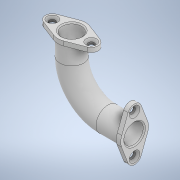
# Autodesk Inventor part: Część14
Saved by Autodesk Inventor 2021 (Build 250183000, 183)
## iProperties
Created: 2023-10-11
Part Number: Część14
Material: Ogólny
Document SubType Name: Modeling
Designer: Jakub
Density: 1 g/cm^3
Appearance: Domyślna
Author: Jakub
Autodesk Inventor part; units mm, degrees
ref_plane "YZ Plane" through (0, 0, 0) normal (1, 0, 0) x (0, 1, 0)
ref_plane "XZ Plane" through (0, 0, 0) normal (0, 1, 0) x (-1, 0, 0)
ref_plane "XY Plane" through (0, 0, 0) normal (0, 0, 1) x (1, 0, 0)
sketch "Szkic1" plane through (0, 0, 0) normal (0, 1, 0) x (-1, 0, 0)
  circle A0 centre (0, 0) radius 25
  line L0 (0, 0) -> (-35, 0)
  line L1 (-35, 0) -> (35, 0)
  circle A1 centre (35, 0) radius 12.5
  circle A2 centre (-35, 0) radius 12.5
  line L2 (35, -12.5) -> (9.6154, -23.0769)
  line L3 (9.6154, -23.0769) -> (39.4603, -11.6771)
  line L4 (9.6154, 23.0769) -> (39.4603, 11.6771)
  line L5 (-9.6154, -23.0769) -> (-39.4603, -11.6771)
  line L6 (-39.4603, 11.6771) -> (-8.2178, 23.6108)
  point P0 (24.1964, 6.2875)
  point P1 (24.1964, -6.2875)
  dimension "d0" = 50
  dimension "d1" = 35
  dimension "d2" = 70
  dimension "d3" = 25
  dimension "d4" = 25
  constraints: 14 end point, 9 point on circle, 5 tangent, 3 centre point, 3 coincident, 1 horizontal, 1 parallel, 1 point on line
  measures "d0" diameter of A0
  measures "d1" distance of L0.start L0.end
  measures "d2" distance of L0.end L1.end
  measures "d3" diameter of A1
  measures "d4" diameter of A2
extrude "Wyciągnięcie proste1" add sketch "Szkic1" along normal blind 8 contours A0 A1 L1 L0 A2 L6 | L4 A1 A0 | A1 A0 | A0 L1 A1 | A0 A2 L6 | A0 A1 L1 | A1 A0 A2 L0 L1 | A2 L0 A0 | A0 A2 | A1 L2 A0 | L3 L2 A1 | L0 A2 A0 | A2 A0 L5
sketch "Szkic2" plane through (0, 8, 0) normal (0, 1, 0) x (1, 0, 0)
  circle A0 centre (0, 0) radius 20
  circle A1 centre (0, 0) radius 17.5
  dimension "d7" = 40
  dimension "d8" = 35
  constraints: 2 centre point, 2 coincident
  measures "d7" diameter of A0
  measures "d8" diameter of A1
extrude "Wyciągnięcie proste2" cut sketch "Szkic2" against normal blind 8 contours A1
chamfer "Faza1" distance 2 angle 45 1 edges at (-17.5, 8, 0)
sketch "Szkic4" plane through (0, 8, 0) normal (0, 1, 0) x (1, 0, 0)
  circle A0 centre (-35, 0) radius 5.5
  circle A1 centre (35, 0) radius 5.5
  point P0 (0, 0)
  dimension "d15" = 11
  dimension "d16" = 11
  constraints: 2 centre point
  measures "d15" diameter of A0
  measures "d16" diameter of A1
extrude "Wyciągnięcie proste3" cut sketch "Szkic4" against normal blind 8
chamfer "Faza2" distance 4 angle 45 2 edges at (-40.5, 8, 0) (29.5, 8, 0)
sketch "Szkic6" plane through (0, 0, 0) normal (0, 0, 1) x (1, 0, 0)
  line L0 (0, 0) -> (-21.5, 0)
  line L1 (9.6154, 0) -> (-9.6154, 0) projected
  line L2 (-21.5, 0) -> (21.5, 0)
  line L3 (8.2178, 0) -> (39.4603, 0) projected
  line L4 (-47.5, 0) -> (-47.5, 8) projected
  line L5 (-47.5, 8) -> (-47.5, -144.5)
  line L6 (21.5, 0) -> (21.5, -32)
  line L7 (21.5, -144.5) -> (-47.5, -144.5)
  line L8 (-47.5, -144.5) -> (105, -144.5)
  line L9 (-21.5, 0) -> (-21.5, -32)
  line L10 (-39.4603, 0) -> (-9.6154, 0) projected
  line L11 (105, -144.5) -> (105, -118.5)
  line L12 (105, -118.5) -> (65, -118.5)
  line L13 (105, -118.5) -> (105, -75.5)
  line L14 (105, -75.5) -> (65, -75.5)
  arc A0 (21.5, -32) -> (65, -75.5) centre (65, -32) ccw
  arc A1 (-21.5, -32) -> (65, -118.5) centre (65, -32) ccw
  point P0 (-21.5, -144.5)
  dimension "d24" = 21.5
  dimension "d25" = 43
  dimension "d26" = 152.5
  dimension "d28" = 152.5
  dimension "d30" = 26
  dimension "d31" = 43
  dimension "d32" = 43.5
  dimension "d33" = 86.5
  constraints: 22 end point, 7 point on line, 4 point on circle, 4 tangent, 2 centre point, 2 collinear, 2 perpendicular, 2 vertical
  measures "d24" distance of L0.start L0.end
  measures "d25" distance of L0.end L2.end
  measures "d26" distance of L5.start L5.end
  measures "d28" distance of L5.end L8.end
  measures "d30" distance of L8.end L11.end
  measures "d31" distance of L11.end L13.end
  measures "d32" radius of A0
  measures "d33" radius of A1
extrude "Wyciągnięcie proste4" [suppressed]
fillet "Zaokrąglenie1" [suppressed]
sketch "Szkic7" plane through (105, -97, 0) normal (1, 0, 0) x (0, 1, 0)
  circle A0 centre (0, 0) radius 25
  line L0 (0, 0) -> (-35, 0)
  line L1 (-35, 0) -> (35, 0)
  circle A1 centre (35, 0) radius 12.5
  circle A2 centre (-35, 0) radius 12.5
  line L2 (35, -12.5) -> (9.6154, -23.0769)
  line L3 (9.6154, -23.0769) -> (39.4603, -11.6771)
  line L4 (9.6154, 23.0769) -> (39.4603, 11.6771)
  line L5 (-9.6154, -23.0769) -> (-39.4603, -11.6771)
  line L6 (-39.4603, 11.6771) -> (-8.2178, 23.6108)
  point P0 (24.1964, 6.2875)
  point P1 (24.1964, -6.2875)
  dimension "d41" = 50
  dimension "d40" = 35
  dimension "d39" = 70
  dimension "d38" = 25
  dimension "d37" = 25
  constraints: 14 end point, 9 point on circle, 5 tangent, 3 centre point, 3 coincident, 1 horizontal, 1 parallel, 1 point on line
  measures "d41" diameter of A0
  measures "d40" distance of L0.start L0.end
  measures "d39" distance of L0.end L1.end
  measures "d38" diameter of A1
  measures "d37" diameter of A2
extrude "Wyciągnięcie proste5" [suppressed]
sketch "Szkic8" plane through (0, 0, 0) normal (0, 0, 1) x (1, 0, 0)
  line L0 (17.5, 0) -> (-17.5, 0) projected
  line L1 (0, 0) -> (17.5, 0)
  line L2 (17.5, 0) -> (-17.5, 0)
  line L3 (-39.4603, 0) -> (-9.6154, 0) projected
  line L4 (47.8218, -144.5) -> (-104.6782, -144.5)
  line L5 (0, 0) -> (-21.5, 0)
  line L6 (-47.5, 0) -> (-47.5, 8) projected
  line L7 (-47.5, 8) -> (-47.5, -144.5)
  line L8 (-17.5, 0) -> (-17.5, -44)
  line L9 (-21.5, 0) -> (-21.5, -32)
  line L10 (9.6154, 0) -> (-9.6154, 0) projected
  line L11 (9.6154, 0) -> (9.6154, -144.5)
  line L12 (17.5, 0) -> (17.5, -36)
  line L13 (-47.5, -144.5) -> (105, -144.5)
  line L14 (105, -144.5) -> (105, -118.5)
  line L15 (105, -118.5) -> (105, -75.5)
  line L16 (105, -75.5) -> (65, -75.5)
  line L17 (105, -97) -> (105, -79.5)
  line L18 (105, -79.5) -> (61, -79.5)
  line L19 (105, -97) -> (105, -114.5)
  line L20 (105, -114.5) -> (9.6154, -114.5)
  line L21 (105, -118.5) -> (65, -118.5)
  line L22 (9.6154, -114.5) -> (53, -114.5)
  line L23 (61, -79.5) -> (53, -79.5)
  line L24 (17.5, -44) -> (17.5, -36)
  line L25 (0, 0) -> (21.5, 0)
  line L26 (8.2178, 0) -> (39.4603, 0) projected
  line L27 (21.5, 0) -> (21.5, -32)
  arc A0 (21.5, -32) -> (65, -75.5) centre (65, -32) ccw
  arc A1 (-21.5, -32) -> (65, -118.5) centre (65, -32) ccw
  line L28 (-21.5, -32) -> (-17.5, -32)
  line L29 (-47.5, -144.5) -> (156.8539, -144.5) construction
  line L30 (3.8353, -93.1647) -> (6.6637, -90.3363)
  line L31 (34.2409, -62.7591) -> (31.4124, -65.5876)
  line L32 (-17.5, -44) -> (-17.5, -32)
  line L33 (65, -114.5) -> (9.6154, -114.5)
  line L34 (53, -79.5) -> (65, -79.5)
  line L35 (17.5, -32) -> (17.5, -44)
  arc A2 (17.5, -32) -> (65, -79.5) centre (65, -32) ccw
  arc A3 (-17.5, -32) -> (65, -114.5) centre (65, -32) ccw
  point P0 (-17.5, -144.5)
  point P1 (-21.5, -144.5)
  point P2 (17.5, -144.5)
  point P3 (-17.5, -114.5)
  dimension "d45" = 35
  dimension "d47" = 152.5
  dimension "d50" = 21.5
  dimension "d51" = 152.5
  dimension "d52" = 26
  dimension "d53" = 43
  dimension "d54" = 17.5
  dimension "d55" = 17.5
  dimension "d59" = 21.5
  dimension "d61" = 86.5
  dimension "d63" = 4
  dimension "d64" = 4
  dimension "d65" = 47.5
  dimension "d66" = 82.5
  constraints: 62 end point, 23 point on line, 13 perpendicular, 10 point on circle, 8 tangent, 4 centre point, 3 collinear, 3 horizontal, 1 midpoint, 1 vertical
  measures "d45" distance of L0.start L2.end
  measures "d47" distance of L4.start L4.end
  measures "d50" distance of L1.start L5.end
  measures "d51" distance of L7.end L13.end
  measures "d52" distance of L13.end L14.end
  measures "d53" distance of L14.end L15.end
  measures "d54" distance of L17.start L17.end
  measures "d55" distance of L17.start L19.end
  measures "d59" distance of L1.start L25.end
  measures "d61" radius of A1
  measures "d63" distance of L30.start L30.end
  measures "d64" distance of L31.start L31.end
  measures "d65" radius of A2
  measures "d66" radius of A3
extrude "Wyciągnięcie proste6" add sketch "Szkic8" along normal mid plane 35 contours L25 L27 A0 L31 A2 L12 | A3 L20 A1 L11 | L11 A1 L30 A3 | L31 A0 L16 L15 L18 A2 | L30 A1 L28 A3 | L20 L15 L21 A1 | L28 L9 L3 L8
sketch "Szkic10" plane through (0, 0, 17.5) normal (0, 0, 1) x (1, 0, 0)
  line L0 (-21.5, 0) -> (-21.5, -32) projected
  line L1 (-21.5, 0) -> (-21.5, -32)
  line L2 (105, -118.5) -> (105, -114.5) projected
  line L3 (105, -118.5) -> (65, -118.5)
  line L4 (105, -75.5) -> (65, -75.5)
  line L5 (21.5, 0) -> (21.5, -32) projected
  line L6 (21.5, 0) -> (21.5, -32)
  line L7 (65, -118.5) -> (105, -118.5) projected
  line L8 (105, -75.5) -> (105, -118.5)
  line L9 (21.5, 0) -> (-21.5, 0)
  line L10 (-39.4603, 0) -> (-9.6154, 0) projected
  arc A0 (-21.5, -32) -> (65, -118.5) centre (65, -32) ccw
  arc A1 (21.5, -32) -> (65, -75.5) centre (65, -32) ccw
  point P0 (0, 0)
  dimension "d71" = 86.5
  dimension "d72" = 43.5
  constraints: 12 end point, 4 point on circle, 4 tangent, 2 centre point, 2 collinear, 2 perpendicular, 1 horizontal, 1 vertical
  measures "d71" radius of A0
  measures "d72" radius of A1
extrude "Wyciągnięcie proste7" add sketch "Szkic10" along normal blind 4
sketch "Szkic13" plane through (0, 0, -17.5) normal (0, 0, -1) x (-1, 0, 0)
  line L0 (9.6154, 0) -> (39.4603, 0) projected
  line L1 (-21.5, 0) -> (-21.5, -32) projected
  line L2 (21.447, 0) -> (-21.5, 0)
  line L3 (-65, -75.5) -> (-105, -75.5) projected
  line L4 (-105, -118.5) -> (-65, -118.5) projected
  line L5 (-105, -75.5) -> (-105, -118.5)
  line L6 (-105, -118.5) -> (-65, -118.5)
  line L7 (21.5, -32) -> (21.5, 0) projected
  line L8 (21.5, 0) -> (21.5, -32)
  line L9 (-21.5, 0) -> (-21.5, -32)
  line L10 (-105, -75.5) -> (-65, -75.5)
  arc A0 (-65, -75.5) -> (-21.5, -32) centre (-65, -32) ccw
  arc A1 (-65, -118.5) -> (21.5, -32) centre (-65, -32) ccw
  point P0 (0, 0)
  point P1 (-21.5, -75.5)
  dimension "d75" = 43.5
  dimension "d76" = 86.5
  constraints: 12 end point, 4 point on circle, 4 point on line, 4 tangent, 2 centre point, 2 perpendicular, 2 vertical, 1 collinear
  measures "d75" radius of A0
  measures "d76" radius of A1
extrude "Wyciągnięcie proste8" add sketch "Szkic13" along normal blind 4
fillet "Zaokrąglenie2" radius 17.5 12 edges at (31.4124, -65.5876, -17.5) (17.5, -16, -17.5) (85, -79.5, -17.5) (6.6637, -90.3363, -17.5) (-17.5, -16, -17.5) (85, -114.5, -17.5) (6.6637, -90.3363, 17.5) (-17.5, -16, 17.5) (85, -114.5, 17.5) (31.4124, -65.5876, 17.5) (17.5, -16, 17.5) (85, -79.5, 17.5)
fillet "Zaokrąglenie3" radius 21.5 12 edges at (85, -75.5, -21.5) (34.2409, -62.7591, -21.5) (21.5, -16, -21.5) (3.8353, -93.1647, -21.5) (-21.5, -16, -21.5) (85, -118.5, -21.5) (3.8353, -93.1647, 21.5) (-21.5, -16, 21.5) (85, -118.5, 21.5) (34.2409, -62.7591, 21.5) (21.5, -16, 21.5) (85, -75.5, 21.5)
sketch "Szkic14" plane through (105, -97, 0) normal (1, 0, 0) x (0, 1, 0)
  circle A0 centre (0, 0) radius 25
  line L0 (0, 0) -> (-35, 0)
  line L1 (-35, 0) -> (35, 0)
  circle A1 centre (35, 0) radius 12.5
  circle A2 centre (-35, 0) radius 12.5
  line L2 (35, -12.5) -> (9.6154, -23.0769)
  line L3 (9.6154, -23.0769) -> (39.4603, -11.6771)
  line L4 (9.6154, 23.0769) -> (39.4603, 11.6771)
  line L5 (-9.6154, -23.0769) -> (-39.4603, -11.6771)
  line L6 (-39.4603, 11.6771) -> (-8.2178, 23.6108)
  point P0 (24.1964, 6.2875)
  point P1 (24.1964, -6.2875)
  dimension "d85" = 50
  dimension "d84" = 35
  dimension "d83" = 70
  dimension "d82" = 25
  dimension "d81" = 25
  constraints: 14 end point, 9 point on circle, 5 tangent, 3 centre point, 3 coincident, 1 horizontal, 1 parallel, 1 point on line
  measures "d85" diameter of A0
  measures "d84" distance of L0.start L0.end
  measures "d83" distance of L0.end L1.end
  measures "d82" diameter of A1
  measures "d81" diameter of A2
extrude "Wyciągnięcie proste9" add sketch "Szkic14" along normal blind 8 contours A0 A1 L1 L0 A2 L6 | L4 A1 A0 | A1 A0 | A0 L1 A1 | A0 A2 L6 | A0 A1 L1 | A1 A0 A2 L0 L1 | A2 L0 A0 | A0 A2 | A1 L2 A0 | L3 L2 A1 | L0 A2 A0 | A2 A0 L5
sketch "Szkic15" plane through (113, -97, 0) normal (1, 0, 0) x (0, 0, -1)
  circle A0 centre (0, 0) radius 17.5
  point P0 (0, 97)
  dimension "d89" = 35
  constraints: 1 centre point
  measures "d89" diameter of A0
extrude "Wyciągnięcie proste10" cut sketch "Szkic15" against normal blind 8
chamfer "Faza3" distance 2 angle 45 1 edges at (113, -97, 17.5)
sketch "Szkic16" plane through (113, -97, 0) normal (1, 0, 0) x (0, 0, -1)
  arc A0 (11.6771, 39.4603) -> (-11.6771, 39.4603) centre (0, 35) ccw projected
  circle A1 centre (0, 35) radius 5.5
  arc A2 (-11.6771, -39.4603) -> (11.6771, -39.4603) centre (0, -35) ccw projected
  circle A3 centre (0, -35) radius 5.5
  point P0 (0, 97)
  dimension "d95" = 11
  dimension "d96" = 11
  constraints: 2 centre point, 2 coincident
  measures "d95" diameter of A1
  measures "d96" diameter of A3
extrude "Wyciągnięcie proste11" cut sketch "Szkic16" against normal blind 8
chamfer "Faza4" distance 4 angle 45 2 edges at (113, -62, 5.5) (113, -132, 5.5)
